Autodesk Inventor part; units mm, degrees
(part 3 of 3)
  arc A102 (20.25, -47.391) -> (18.25, -45.391) centre (18.25, -47.391) ccw
  arc A103 (10.75, -52.891) -> (12.75, -54.891) centre (12.75, -52.891) ccw
  line L329 (-20.25, -16.391) -> (-20.25, -21.891)
  line L330 (-18.2, -20.6998) -> (-18.2, -17.5822)
  arc A104 (-18.25, -14.391) -> (-20.25, -16.391) centre (-18.25, -16.391) ccw
  line L331 (-15.5, -22.2587) -> (-18.2, -20.6998)
  line L332 (-18.2, -17.5822) -> (-15.5, -16.0233)
  line L333 (-12.8, -17.5822) -> (-12.8, -20.6998)
  line L334 (-12.8, -20.6998) -> (-15.5, -22.2587)
  line L335 (-18.25, -23.891) -> (-12.75, -23.891)
  line L336 (-15.5, -16.0233) -> (-12.8, -17.5822)
  line L337 (-12.75, -14.391) -> (-18.25, -14.391)
  line L338 (-10.75, -21.891) -> (-10.75, -16.391)
  arc A105 (-12.75, -23.891) -> (-10.75, -21.891) centre (-12.75, -21.891) ccw
  line L339 (-20.25, -23.891) -> (-10.75, -14.391) construction
  line L340 (-10.75, -23.891) -> (-20.25, -14.391) construction
  arc A106 (-10.75, -16.391) -> (-12.75, -14.391) centre (-12.75, -16.391) ccw
  arc A107 (-20.25, -21.891) -> (-18.25, -23.891) centre (-18.25, -21.891) ccw
  circle A108 centre (-114.25, 78.75) radius 5.11
  circle A109 centre (-114.25, -78.75) radius 5.11
  arc A110 (-100.25, 84.75) -> (-102.25, 86.75) centre (-102.25, 84.75) ccw
  arc A111 (-102.25, 70.75) -> (-100.25, 72.75) centre (-102.25, 72.75) ccw
  arc A112 (-100.25, -72.75) -> (-102.25, -70.75) centre (-102.25, -72.75) ccw
  arc A113 (-102.25, -86.75) -> (-100.25, -84.75) centre (-102.25, -84.75) ccw
  arc A114 (-80.25, -100.25) -> (-90.25, -90.25) centre (-90.25, -100.25) ccw
  arc A115 (-116.25, -90.25) -> (-126.25, -100.25) centre (-116.25, -100.25) ccw
  line L341 (-80.25, 101.25) -> (-80.25, 100.25)
  line L342 (-90.25, 90.25) -> (-116.25, 90.25)
  arc A116 (-90.25, 90.25) -> (-80.25, 100.25) centre (-90.25, 100.25) ccw
  line L343 (-126.25, 101.25) -> (-126.25, 100.25)
  arc A117 (-126.25, 100.25) -> (-116.25, 90.25) centre (-116.25, 100.25) ccw
  line L344 (154.75, 100.25) -> (142.75, 100.25)
  line L345 (140.75, 100.25) -> (140.75, 114.25)
  line L346 (142.75, 116.25) -> (154.75, 116.25)
  line L347 (156.75, 114.25) -> (156.75, 102.25)
  line L348 (140.75, 116.25) -> (136.75, 116.25)
  line L349 (134.75, 114.25) -> (134.75, 102.25)
  line L350 (136.75, 100.25) -> (140.75, 100.25)
  line L351 (140.75, 102.25) -> (140.75, 116.25)
  circle A118 centre (148.75, 108.25) radius 3
  line L352 (145.8921, 103.3) -> (143.0342, 108.25)
  line L353 (143.0342, 108.25) -> (145.8921, 113.2)
  line L354 (145.8921, 113.2) -> (151.6079, 113.2)
  line L355 (151.6079, 113.2) -> (154.4658, 108.25)
  line L356 (154.4658, 108.25) -> (151.6079, 103.3)
  line L357 (151.6079, 103.3) -> (145.8921, 103.3)
  arc A119 (134.75, 102.25) -> (136.75, 100.25) centre (136.75, 102.25) ccw
  arc A120 (136.75, 116.25) -> (134.75, 114.25) centre (136.75, 114.25) ccw
  arc A121 (142.75, 116.25) -> (140.75, 114.25) centre (142.75, 114.25) ccw
  arc A122 (140.75, 102.25) -> (142.75, 100.25) centre (142.75, 102.25) ccw
  arc A123 (154.75, 100.25) -> (156.75, 102.25) centre (154.75, 102.25) ccw
  arc A124 (156.75, 114.25) -> (154.75, 116.25) centre (154.75, 114.25) ccw
  line L358 (142.75, 100.25) -> (140.75, 100.25)
  line L359 (142.75, 116.25) -> (140.75, 116.25)
  line L360 (140.75, -116.25) -> (136.75, -116.25)
  line L361 (134.75, -114.25) -> (134.75, -102.25)
  line L362 (142.75, -116.25) -> (140.75, -116.25)
  arc A125 (134.75, -114.25) -> (136.75, -116.25) centre (136.75, -114.25) ccw
  arc A126 (156.75, -102.25) -> (154.75, -100.25) centre (154.75, -102.25) ccw
  line L363 (145.8921, -113.2) -> (151.6079, -113.2)
  line L364 (151.6079, -103.3) -> (145.8921, -103.3)
  circle A127 centre (148.75, -108.25) radius 3
  line L365 (143.0342, -108.25) -> (145.8921, -113.2)
  line L366 (142.75, -116.25) -> (154.75, -116.25)
  line L367 (140.75, -102.25) -> (140.75, -116.25)
  arc A128 (140.75, -114.25) -> (142.75, -116.25) centre (142.75, -114.25) ccw
  line L368 (140.75, -100.25) -> (140.75, -114.25)
  line L369 (145.8921, -103.3) -> (143.0342, -108.25)
  arc A129 (142.75, -100.25) -> (140.75, -102.25) centre (142.75, -102.25) ccw
  line L370 (154.75, -100.25) -> (142.75, -100.25)
  line L371 (154.4658, -108.25) -> (151.6079, -103.3)
  line L372 (151.6079, -113.2) -> (154.4658, -108.25)
  line L373 (156.75, -114.25) -> (156.75, -102.25)
  arc A130 (154.75, -116.25) -> (156.75, -114.25) centre (154.75, -114.25) ccw
  arc A131 (136.75, -100.25) -> (134.75, -102.25) centre (136.75, -102.25) ccw
  line L374 (136.75, -100.25) -> (140.75, -100.25)
  line L375 (142.75, -100.25) -> (140.75, -100.25)
  circle A132 centre (148.75, -108.25) radius 5.11
  circle A133 centre (148.75, 108.25) radius 5.11
  point P0 (-45.4663, -26.25)
  point P1 (42.5123, 3.7193)
  point P2 (34, 11)
  point P3 (31.5, 0)
  point P4 (34, -11)
  point P5 (0, 122.25)
  point P6 (0, -122.25)
  point P7 (-122.25, 0)
  point P8 (-45.4663, -26.25)
  point P9 (42.4707, -4.4638)
  point P10 (31, 14.5)
  point P11 (112.25, -89.75)
  point P12 (137.25, -124.75)
  point P13 (54.5596, -31.5)
  point P14 (45.4663, -26.25)
  point P15 (0, 63)
  point P16 (0, 52.5)
  point P17 (-126.25, 95.75)
  point P18 (-100.25, 86.75)
  point P19 (-100.25, -70.75)
  point P20 (-9.7, 47)
  point P21 (-35.8532, -31.9004)
  point P22 (-38.7032, -26.9641)
  point P23 (-38.7032, -26.9641)
  point P24 (-42.7032, -20.0359)
  point P25 (-38.7032, -26.9641)
  point P26 (-42.7032, -20.0359)
  point P27 (45.5532, -15.0996)
  point P28 (42.7032, -20.0359)
  point P29 (42.7032, -20.0359)
  point P30 (38.7032, -26.9641)
  point P31 (42.7032, -20.0359)
  point P32 (38.7032, -26.9641)
  point P33 (-15.5, -19.141)
  point P34 (-80.25, 90.25)
  point P35 (-126.25, 90.25)
  point P36 (156.75, 108.25)
  point P37 (148.75, 100.25)
  point P38 (148.75, -100.25)
  point P39 (156.75, -108.25)
  point P40 (0, 122.25)
  point P41 (0, -122.25)
  dimension "d434" = 236.532
  dimension "d435" = 238.5
  dimension "d436" = 290
  dimension "d437" = 3
  dimension "d438" = 6
  dimension "d439" = 4
  dimension "d440" = 208
  dimension "d441" = 220.735
  dimension "d442" = 126
  dimension "d443" = 4
  dimension "d444" = 2
  dimension "d445" = 2
  dimension "d446" = 2
  dimension "d447" = 25
  dimension "d448" = 46
  dimension "d449" = 25
  dimension "d450" = 10
  dimension "d451" = 10
  dimension "d452" = 110.851
  dimension "d453" = 5
  dimension "d454" = 6
  dimension "d455" = 41.569
  dimension "d456" = 12
  dimension "d457" = 35
  dimension "d458" = 6
  dimension "d459" = 12.5
  dimension "d460" = 5
  dimension "d461" = 7
  dimension "d462" = 6
  dimension "d463" = 10
  dimension "d464" = 10
  dimension "d465" = 58
  dimension "d466" = 45
  dimension "d467" = 15
  dimension "d468" = 40
  dimension "d469" = 25
  dimension "d470" = 15
  dimension "d471" = 110
  dimension "d472" = 70
  dimension "d473" = 50
  dimension "d474" = 63
  dimension "d475" = 3
  dimension "d476" = 1.5
  dimension "d478" = 4
  dimension "d479" = 18
  dimension "d480" = 15
  dimension "d481" = 3
  dimension "d482" = 2
  dimension "d483" = 2
  dimension "d484" = 5
  dimension "d485" = 236
  dimension "d486" = 42.3
  dimension "d487" = 31
  dimension "d488" = 31
  dimension "d489" = 33
  dimension "d490" = 30
  dimension "d491" = 5
  dimension "d492" = 22
  dimension "d493" = 2
  dimension "d494" = 2
  dimension "d495" = 2
  dimension "d496" = 2
  dimension "d497" = 360
  dimension "d498" = 1.5
  constraints: 756 end point, 179 point on circle, 146 point on line, 137 tangent, 129 centre point, 72 symmetric about line, 61 parallel, 49 equal radius, 49 perpendicular, 48 midpoint, 40 coincident, 39 horizontal, 26 equal length, 26 vertical alignment, 19 vertical, 14 horizontal alignment, 3 collinear, 457 other
  measures "d434" diameter of A6
  measures "d435" diameter of A7
  measures "d436" distance of L38.start L38.end
  measures "d438" distance between parallel lines of L4 L3
  measures "d439" distance between parallel lines of L38 L33
  measures "d440" diameter of A4
  measures "d441" diameter of A5
  measures "d442" diameter of A3
  measures "d443" distance from line of point (-122.25, 0) L31
  measures "d444" distance between parallel lines of L38 L2
  measures "d445" distance between parallel lines of L31 L47
  measures "d446" distance between parallel lines of L35 L41
  measures "d447" distance of L38.start L343.start
  measures "d448" distance of L38.start L100.start
  measures "d449" distance of L31.start L87.end
  measures "d450" diameter of A29
  measures "d451" diameter of A15
  measures "d452" diameter of A2
  measures "d453" angle of L81 L82
  measures "d454" angle of L81 L80
  measures "d455" diameter of A1
  measures "d456" distance of L21.start L7.start
  measures "d457" distance of L7.start L8.start
  measures "d458" distance of L12.start L14.end
  measures "d459" distance of L14.end L13.start
  measures "d460" distance between parallel lines of L7 L18
  measures "d461" distance of L23.end L25.start
  measures "d462" distance of L25.start L25.end
  measures "d463" distance from line of L101 A29.centre
  measures "d464" distance from line of L38 A29.centre
  measures "d465" distance between parallel lines of L38 L32
  measures "d466" distance from line of L39 A21.centre
  measures "d467" diameter of A23
  measures "d468" vertical distance of A4.centre A23.centre
  measures "d469" horizontal distance of A4.centre A23.centre
  measures "d470" diameter of A22
  measures "d471" distance of L84.start L84.end
  measures "d472" distance of L91.start L91.end
  measures "d473" distance of L91.end L92.start
  measures "d475" diameter of A28
  measures "d476" distance between parallel lines of L35 L95
  measures "d478" distance edge to line of A10 L51
  measures "d479" distance of L51.end L59.end
  measures "d480" distance of L59.end L52.start
  measures "d481" diameter of A13
  measures "d482" distance edge to line of A13 L0
  measures "d483" distance edge to line of A13 L60
  measures "d484" diameter of A10
  measures "d485" distance of L32.start L32.end
  measures "d486" distance of L107.start L110.start
  measures "d487" distance of A30.centre A33.centre
  measures "d488" distance of A31.centre A30.centre
  measures "d489" distance of L112.start L111.start
  measures "d490" distance between parallel lines of L49 L71
  measures "d491" distance between parallel lines of L114 L49
  measures "d492" distance of L22.end L18.start
  measures "d493" distance of L117.start L59.end
  measures "d494" distance of L0.start L59.end
  measures "d495" distance of L53.start L52.start
  measures "d496" distance of L0.end L52.start
  measures "d498" distance between parallel lines of L39 L91
extrude "Выдавливание34" cut sketch "Эскиз4" against normal blind 2 contours A5 bodies 2
extrude "Выдавливание35" cut sketch "Эскиз4" against normal blind 2.5 contours L2 L85 L38 L4 | L2 L3 L38 L85 | L38 L85 A8 L4 | L38 L3 A8 L85 | A8 L85 A7 L58 | A8 L43 A7 L85 | A8 L58 L31 L57 | L58 A7 L43 A8 | A8 L48 L31 L58 | L31 L58 L47 L57 | L31 L48 L47 L58 | L42 L35 L43 A8 | A8 L43 L35 L40 | L42 L41 L43 L35 | L35 L43 L41 L40 bodies 2
ref_plane "РабПлоскость2" through (-130.25, 0, 0) normal (0, 1, 0) x (1, 0, 0)
split body "Разделение1" result two bodies by plane through (-130.25, 0, 0) normal (0, 1, 0) bodies 1 first body at (37.0535, 70.7677, -9.5)
split body "Разделение2" result two bodies by plane through (-130.25, 0, 0) normal (0, 1, 0) bodies 2 first body at (9.2269, 93.663, 0.5)
sketch "Эскиз5" plane through (0, 0, 4) normal (0, 0, 1) x (1, 0, 0)
  circle A0 centre (0, -95.25) radius 1.5
  line L0 (-130.25, -130.25) -> (167.75, -130.25) projected
  circle A1 centre (97.975, -10) radius 1.5
  line L1 (104, 0) -> (91.95, 0) projected
  circle A2 centre (-97.975, -10) radius 1.5
  line L2 (-91.95, 0) -> (-104, 0) projected
  point P0 (0, 0)
  point P1 (97.975, 0)
  point P2 (-97.975, 0)
  dimension "d587" = 3
  dimension "d588" = 35
  dimension "d603" = 3
  dimension "d604" = 10
  dimension "d605" = 3
  dimension "d606" = 10
  constraints: 3 centre point, 3 vertical alignment, 2 midpoint
  measures "d587" diameter of A0
  measures "d588" distance from line of L0 A0.centre
  measures "d603" diameter of A1
  measures "d604" distance from line of A1.centre L1
  measures "d605" diameter of A2
  measures "d606" distance from line of A2.centre L2
extrude "Выдавливание37" cut sketch "Эскиз5" against normal through all bodies 6
sketch "Эскиз6" plane through (0, 0, 4) normal (0, 0, 1) x (1, 0, 0)
  circle A0 centre (0, 0) radius 78.0765 construction
  circle A1 centre (55.2084, 55.2084) radius 5 construction
  line L0 (0, 0) -> (55.2084, 55.2084) construction
  line L1 (72.05, 0) -> (-72.05, 0) projected
  line L2 (55.1731, 53.0517) -> (44.5665, 42.4451)
  line L3 (53.0517, 55.1731) -> (55.1731, 53.0517)
  line L4 (42.4451, 44.5665) -> (53.0517, 55.1731)
  line L5 (55.5832, 52.6416) -> (52.6416, 55.5832)
  line L6 (52.6416, 55.5832) -> (54.8337, 57.7752)
  line L7 (54.8337, 57.7752) -> (57.7752, 54.8337)
  line L8 (57.7752, 54.8337) -> (52.6416, 55.5832) construction
  line L9 (54.8337, 57.7752) -> (55.5832, 52.6416) construction
  line L10 (57.7752, 54.8337) -> (55.5832, 52.6416)
  line L11 (44.5665, 42.4451) -> (42.4451, 44.5665)
  line L12 (56.3044, 56.3044) -> (43.5058, 43.5058) construction
  line L13 (51.3547, 61.2542) -> (38.5561, 48.4556)
  line L14 (48.4556, 38.5561) -> (61.2542, 51.3547)
  arc A2 (61.2542, 51.3547) -> (51.3547, 61.2542) centre (56.3044, 56.3044) ccw
  arc A3 (38.5561, 48.4556) -> (48.4556, 38.5561) centre (43.5058, 43.5058) ccw
  line L15 (53.0517, 55.1731) -> (47.7484, 49.8698)
  line L16 (55.1731, 53.0517) -> (49.8698, 47.7484)
  line L17 (50.4001, 52.5214) -> (39.5498, 47.4618)
  line L18 (52.5214, 50.4001) -> (47.4618, 39.5498)
  arc A4 (39.5498, 47.4618) -> (47.4618, 39.5498) centre (54.3749, 54.3749) ccw
  line L19 (52.5214, 50.4001) -> (50.4001, 52.5214)
  line L20 (39.5498, 47.4618) -> (42.4451, 44.5665) construction
  point P0 (54.1124, 54.1124)
  point P1 (49.9051, 49.9051)
  dimension "d591" = 156.153
  dimension "d592" = 10
  dimension "d593" = 45
  dimension "d594" = 4.06
  dimension "d595" = 3
  dimension "d596" = 3
  dimension "d597" = 15
  dimension "d598" = 14
  dimension "d599" = 20
  dimension "d600" = 20
  constraints: 42 end point, 10 midpoint, 8 parallel, 6 coincident, 6 point on circle, 4 centre point, 4 tangent, 3 perpendicular, 2 line through centre, 2 point on line, 3 other
  measures "d592" diameter of A1
  measures "d593" angle of L1 L0
  measures "d596" distance of L2.end L4.start
  measures "d597" distance of L16.start L2.end
  measures "d598" diameter of A3
  measures "d599" angle of L2 L18
  measures "d600" angle of L4 L17
extrude "Выдавливание38" cut sketch "Эскиз6" against normal blind 10 contours L2 L19 L4 L3 | L3 L5 L6 L7 L10 | L18 A4 L17 L4 L11 L2 | L2 L11 L4 L19 | A2 L14 A3 L13 bodies 5
sketch "Эскиз8" plane through (0, 0, 4) normal (0, 0, 1) x (1, 0, 0)
  circle A0 centre (97.975, 10) radius 1.5
  line L0 (104, 0) -> (91.95, 0) projected
  circle A1 centre (-97.975, 10) radius 1.5
  line L1 (-91.95, 0) -> (-104, 0) projected
  circle A2 centre (0, 95.25) radius 1.5
  line L2 (167.75, 130.25) -> (-130.25, 130.25) projected
  line L3 (-3, 128.25) -> (3, 128.25) projected
  circle A3 centre (-40.25, 40.25) radius 1.5
  line L4 (-130.25, 130.25) -> (-130.25, 0) projected
  point P0 (0, 0)
  point P1 (97.975, 0)
  point P2 (-97.975, 0)
  point P3 (0, 128.25)
  dimension "d607" = 3
  dimension "d608" = 10
  dimension "d609" = 3
  dimension "d610" = 10
  dimension "d611" = 3
  dimension "d612" = 35
  dimension "d613" = 3
  dimension "d614" = 90
  dimension "d615" = 90
  constraints: 4 centre point, 3 midpoint, 3 vertical alignment
  measures "d607" diameter of A0
  measures "d608" distance from line of A0.centre L0
  measures "d609" diameter of A1
  measures "d610" distance from line of L1 A1.centre
  measures "d611" diameter of A2
  measures "d612" distance from line of L2 A2.centre
  measures "d613" diameter of A3
  measures "d614" distance from line of L2 A3.centre
  measures "d615" distance from line of L4 A3.centre
extrude "Выдавливание39" cut sketch "Эскиз8" against normal through all contours A0 | A1 | A3 bodies 5
sketch "Эскиз9" plane through (0, 0, 0) normal (0, 0, 1) x (1, 0, 0)
  circle A0 centre (-114.75, -95.75) radius 1.5 projected
  circle A1 centre (-91.75, -95.75) radius 1.5 projected
  circle A2 centre (-42.7032, -20.0359) radius 1.5 projected
  circle A3 centre (-38.7032, -26.9641) radius 1.5 projected
  circle A4 centre (-15.5, -50.141) radius 1.5 projected
  circle A5 centre (-15.5, -19.141) radius 1.5 projected
  circle A6 centre (15.5, -50.141) radius 1.5 projected
  circle A7 centre (15.5, -19.141) radius 1.5 projected
  circle A8 centre (31.5, -13.5) radius 1.5 projected
  circle A9 centre (42.7032, -20.0359) radius 1.5 projected
  circle A10 centre (38.7032, -26.9641) radius 1.5 projected
  circle A11 centre (31.5, 13.5) radius 1.5 projected
  circle A12 centre (114.75, -56.75) radius 1.5 projected
  circle A13 centre (114.75, -122.75) radius 1.5 projected
  circle A14 centre (159.75, -122.75) radius 1.5 projected
  circle A15 centre (159.75, -56.75) radius 1.5 projected
  circle A16 centre (4, 47) radius 1.5 projected
  circle A17 centre (-4, 47) radius 1.5 projected
  circle A18 centre (-114.75, 95.75) radius 1.5 projected
  circle A19 centre (-91.75, 95.75) radius 1.5 projected
  circle A20 centre (-114.75, -95.75) radius 2.25
  circle A21 centre (-91.75, -95.75) radius 2.25
  circle A22 centre (-42.7032, -20.0359) radius 2.25
  circle A23 centre (-38.7032, -26.9641) radius 2.25
  circle A24 centre (-15.5, -50.141) radius 2.25
  circle A25 centre (-15.5, -19.141) radius 2.25
  circle A26 centre (15.5, -50.141) radius 2.25
  circle A27 centre (15.5, -19.141) radius 2.25
  circle A28 centre (31.5, -13.5) radius 2.25
  circle A29 centre (42.7032, -20.0359) radius 2.25
  circle A30 centre (38.7032, -26.9641) radius 2.25
  circle A31 centre (31.5, 13.5) radius 2.25
  circle A32 centre (4, 47) radius 2.25
  circle A33 centre (-4, 47) radius 2.25
  circle A34 centre (-114.75, 95.75) radius 2.25
  circle A35 centre (-91.75, 95.75) radius 2.25
  circle A36 centre (114.75, -56.75) radius 2.25
  circle A37 centre (159.75, -56.75) radius 2.25
  circle A38 centre (159.75, -122.75) radius 2.25
  circle A39 centre (114.75, -122.75) radius 2.25
  point P0 (0, 0)
  dimension "d618" = 4.5
  constraints: 20 centre point, 19 equal radius
  measures "d618" diameter of A20
extrude "Выдавливание40" cut sketch "Эскиз9" against normal up to surface (6 mm away) contours A0 | A1 | A2 | A3 | A4 | A5 | A6 | A7 | A8 | A9 | A10 | A11 | A12 | A13 | A14 | A15 | A16 | A17 | A18 | A19 | A20 | A21 | A22 | A23 | A24 | A25 | A26 | A27 | A28 | A29 | A30 | A31 | A32 | A33 | A34 | A35 | A36 | A37 | A38 | A39 bodies 4 3
